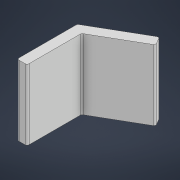
# Autodesk Inventor part: Лепесток БСП
Saved by Autodesk Inventor 2022 (Build 260153000, 153)
## iProperties
Created: 2023-02-18
Part Number: Лепесток БСП
Material: Типовые
Document SubType Name: Modeling
Designer: Глеб
Density: 1 g/cm^3
Appearance: По умолчанию
Author: Глеб
Autodesk Inventor part; units mm, degrees
ref_plane "YZ Plane" through (0, 0, 0) normal (1, 0, 0) x (0, 1, 0)
ref_plane "XZ Plane" through (0, 0, 0) normal (0, 1, 0) x (-1, 0, 0)
ref_plane "XY Plane" through (0, 0, 0) normal (0, 0, 1) x (1, 0, 0)
sketch "Эскиз1" plane through (0, 0, 0) normal (0, 1, 0) x (-1, 0, 0)
  line L0 (16.3923, 0) -> (-63.3538, 0) construction
  line L1 (5, 30) -> (-5, 30)
  line L2 (5, -30) -> (5, 30)
  line L3 (5, -30) -> (-46.9615, -60)
  line L4 (-46.9615, -60) -> (-51.9615, -51.3397)
  line L5 (-51.9615, -51.3397) -> (-5, -24.2265)
  line L6 (-5, -24.2265) -> (-5, 30)
  line L7 (0, -78) -> (0, 48) construction
  point P0 (0, 0)
  dimension "d13" = 60
  dimension "d16" = 10
  dimension "d17" = 10
  dimension "d18" = 60
  dimension "d19" = 120
  constraints: 12 end point, 2 perpendicular, 1 horizontal, 1 parallel, 1 symmetric about line
  measures "d13" distance from line of L2.start L1
  measures "d16" distance between parallel lines of L5 L3
  measures "d17" distance between parallel lines of L6 L2
  measures "d18" distance from line of L4 L2.start
  measures "d19" angle of L5 L6
extrude "Выдавливание1" add sketch "Эскиз1" along normal blind 70
fillet "Сопряжение1" radius 2 6 edges at (-5, 35, 30) (5, 35, 30) (-5, 35, -30) (51.9615, 35, -51.3397) (46.9615, 35, -60) (5, 35, -24.2265)
sketch "Эскиз7" plane through (0, 0, 0) normal (0, -1, 0) x (1, 0, 0)
  line L0 (-3, 30) -> (3, 30) projected
  line L1 (5, 28) -> (5, -23.0718) projected
  line L2 (6, -24.8038) -> (50.2295, -50.3397) projected
  line L3 (50.9615, -53.0718) -> (47.9615, -58.2679) projected
  point P0 (0, 0)
  point P1 (0, 25)
  point P2 (45.1314, -53.1699)
  dimension "d21" = 5
  dimension "d22" = 5
  dimension "d23" = 5
  dimension "d24" = 5
  measures "d21" distance from line of L0 point (0, 25)
  measures "d22" distance from line of L1 point (0, 25)
  measures "d23" distance from line of L2 point (45.131, -53.17)
  measures "d24" distance from line of L3 point (45.131, -53.17)
hole "Отверстие1" at (0, 0, 25) at (45.1314, 0, -53.1699) direction (0, 1, 0) diameter 3 depth 60 tip angle 118
equation "\"d22\" = d21"
equation "\"d23\" = d24"
equation "\"d24\" = d21"
